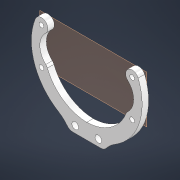
# Autodesk Inventor part: mount
Saved by Autodesk Inventor 2021 (Build 250183000, 183)
## iProperties
Created: 2021-01-20
Part Number: mount
Material: ABS Plastic
Document SubType Name: Modeling
Designer: User
Density: 1.06 g/cm^3
Appearance: Smooth - White
Author: User
Autodesk Inventor part; units mm, degrees
ref_plane "YZ Plane" through (0, 0, 0) normal (1, 0, 0) x (0, 1, 0)
ref_plane "XZ Plane" through (0, 0, 0) normal (0, 1, 0) x (-1, 0, 0)
ref_plane "XY Plane" through (0, 0, 0) normal (0, 0, 1) x (1, 0, 0)
ref_plane "Work Plane1" through (0, 0, 0) normal (0, 0, 1) x (1, 0, 0)
sketch "Sketch1" plane through (0, 0, 0) normal (0, 0, 1) x (1, 0, 0)
  line L0 (22.5, 10) -> (22.5, -10) construction
  line L1 (-22.5, 10) -> (22.5, 10) construction
  line L2 (-22.5, -10) -> (-22.5, 10) construction
  line L3 (22.5, -10) -> (-22.5, -10) construction
  circle A0 centre (-13.1, -5.1) radius 0.75 construction
  circle A1 centre (-13.1, 5.1) radius 0.75 construction
  circle A2 centre (-2.44, 7) radius 0.5 construction
  circle A3 centre (-3.81, -8) radius 0.5 construction
  circle A4 centre (-1.27, -8) radius 0.5 construction
  circle A5 centre (1.27, -8) radius 0.5 construction
  circle A6 centre (-21, -8.5) radius 1 projected
  circle A7 centre (21, -8.5) radius 1 projected
  circle A8 centre (-21, 8.5) radius 1 projected
  circle A9 centre (21, 8.5) radius 1 projected
  circle A10 centre (3.81, -8) radius 0.5 construction
  circle A11 centre (2.44, 7) radius 0.5 construction
  circle A12 centre (13.1, 5.1) radius 0.75 construction
  circle A13 centre (13.1, -5.1) radius 0.75 construction
  circle A14 centre (-13.1789, 0.0006) radius 7.9502 construction
  circle A15 centre (13.1, 0) radius 7.9502 construction
  circle A16 centre (-21, 8.5) radius 3
  circle A17 centre (-21, -8.5) radius 3
  arc A18 (-18.9688, 6.2923) -> (-18.9688, -6.2923) centre (-13.1795, 0) ccw
  arc A19 (-23.7876, 9.6087) -> (-23.7876, -9.6087) centre (0.3717, 0) ccw
  line L4 (0, 10) -> (0, -10) construction
  line L5 (-6.9, -24) -> (6.9, -24) construction
  line L6 (-5.35, -25.55) -> (5.35, -25.55) construction
  line L7 (5.35, -22.45) -> (-5.35, -22.45) construction
  arc A20 (-5.35, -22.45) -> (-5.35, -25.55) centre (-5.35, -24) ccw construction
  arc A21 (5.35, -25.55) -> (5.35, -22.45) centre (5.35, -24) ccw construction
  arc A22 (-23.7876, -9.6087) -> (-13.0267, -22.2819) centre (0.3717, 0) ccw
  line L8 (-9.6283, -24) -> (9.6283, -24) construction
  line L9 (-6.5283, -27.1) -> (6.5283, -27.1)
  line L10 (6.5283, -20.9) -> (-6.5283, -20.9) construction
  arc A23 (-8.9873, -25.8877) -> (-6.5283, -27.1) centre (-6.5283, -24) ccw
  arc A24 (6.5283, -27.1) -> (6.5283, -20.9) centre (6.5283, -24) ccw construction
  circle A25 centre (-5.35, -24) radius 1.55
  circle A26 centre (5.35, -24) radius 1.55
  arc A27 (-18.2124, -7.3913) -> (0, -19.9965) centre (0.3717, 0) ccw
  arc A28 (-8.9873, -25.8877) -> (-13.0267, -22.2819) centre (-20.5173, -34.7387) ccw
  line L11 (6.5283, -27.1) -> (-6.5283, -27.1)
  circle A29 centre (21, 8.5) radius 3
  circle A30 centre (21, -8.5) radius 3
  arc A31 (18.9688, -6.2923) -> (18.9688, 6.2923) centre (13.1795, 0) ccw
  arc A32 (23.7876, -9.6087) -> (23.7876, 9.6087) centre (-0.3717, 0) ccw
  arc A33 (13.0267, -22.2819) -> (23.7876, -9.6087) centre (-0.3717, 0) ccw
  arc A34 (6.5283, -27.1) -> (8.9873, -25.8877) centre (6.5283, -24) ccw
  arc A35 (0, -19.9965) -> (18.2124, -7.3913) centre (-0.3717, 0) ccw
  arc A36 (13.0267, -22.2819) -> (8.9873, -25.8877) centre (20.5173, -34.7387) ccw
  circle A37 centre (-21, 8.5) radius 1.1
  circle A38 centre (-21, -8.5) radius 1.1
  circle A39 centre (21, 8.5) radius 1.1
  circle A40 centre (21, -8.5) radius 1.1
  point P0 (0, 0)
  point P1 (0, -24)
  point P2 (0, 0)
  point P3 (0, -24)
  point P4 (-7.8991, -26.7804)
  point P5 (6.5283, -27.1)
  dimension "d0" = 6
  dimension "d11" = 17
  dimension "d16" = 15.9004
  dimension "d17" = 8.5503
  dimension "d19" = 8.5503
  dimension "d21" = 13.8
  dimension "d22" = 3.1
  dimension "d24" = 9.6283
  dimension "d25" = 19.2566
  dimension "d26" = 6.2
  dimension "d29" = 14.5355
  dimension "d32" = 24
  dimension "d33" = 26
  dimension "d34" = 0.1
  dimension "d35" = 0.1
  dimension "d36" = 0.1
  dimension "d37" = 0.1
  constraints: 47 point on circle, 23 centre point, 20 end point, 18 symmetric about line, 16 tangent, 7 coincident, 5 midpoint, 5 point on line, 4 vertical alignment, 2 concentric, 2 horizontal, 2 parallel, 1 horizontal alignment, 1 vertical, 14 other
  measures "d0" diameter of A16
  measures "d11" distance of A16.centre A17.centre
  measures "d16" diameter of A14
  measures "d17" radius of A18
  measures "d19" distance of A14.centre A16.start
  measures "d21" distance of L5.end L5.start
  measures "d22" distance between parallel lines of L6 L7
  measures "d24" distance of point (0, -24) L8.start
  measures "d25" distance of L8.end L8.start
  measures "d26" distance between parallel lines of L10 L9
  measures "d29" radius of A28
  measures "d32" distance of point (0, 0) point (0, -24)
  measures "d33" radius of A19
  measures "d34" radial gap between concentric circles of A8 A37
  measures "d35" radial gap between concentric circles of A7 A40
  measures "d36" radial gap between concentric circles of A9 A39
  measures "d37" radial gap between concentric circles of A6 A38
extrude "Extrusion1" add sketch "Sketch1" along normal blind 3 contours A16 | A16 A18 A17 A19 | A17 | A17 A27 A35 A30 A33 A36 A34 L9 A23 A28 A22 | A30 | A31 A29 A32 A30 | A29
equation "\"d17\" = d19"
equation "\"d25\" = 2 * d24"
equation "\"d26\" = 2 * d22"
body "Solid1"
